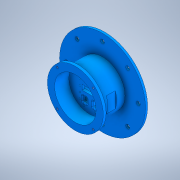
# Autodesk Inventor part: B-02
Saved by Autodesk Inventor 2021 (Build 250183000, 183)
## iProperties
Created: 2021-10-04
Part Number: B-02
Material: PETG
Document SubType Name: Modeling
Designer: Alcatraz
Density: 1.27 g/cm^3
Appearance: Genérico
Author: Alcatraz
Autodesk Inventor part; units mm, degrees
sketch "Boceto1" plane through (0, 0, 0) normal (0, 0, 1) x (1, 0, 0)
  line L0 (-16, -25) -> (16, -25)
  line L1 (16, -25) -> (16, 25)
  line L2 (16, 25) -> (-16, 25)
  line L3 (-16, 25) -> (-16, -25)
  line L4 (-16, -25) -> (16, 25) construction
  line L5 (16, -25) -> (-16, 25) construction
  circle A0 centre (0, 13.5) radius 6
  circle A1 centre (-8, -22.5) radius 1.1
  circle A2 centre (8, -22.5) radius 1.1
  circle A3 centre (13.5, -17) radius 1.1
  circle A4 centre (-13.5, -17) radius 1.1
  circle A5 centre (-13.5, -9) radius 1.1
  circle A6 centre (-13.5, -1) radius 1.1
  circle A7 centre (-13.5, 7) radius 1.1
  circle A8 centre (13.5, 7) radius 1.1
  circle A9 centre (13.5, -1) radius 1.1
  circle A10 centre (13.5, -9) radius 1.1
  line L6 (0, 1.85) -> (10.5, 1.85)
  line L7 (10.5, 1.85) -> (10.5, -5.15)
  line L8 (10.5, -5.15) -> (-10.5, -5.15)
  line L9 (-10.5, -5.15) -> (-10.5, 1.85)
  line L10 (-10.5, 1.85) -> (0, 1.85)
  line L11 (0, -25) -> (0, -15.266)
  line L12 (-7, -11.666) -> (-4.8, -11.666)
  line L13 (-7, -11.666) -> (-9.2, -11.666)
  line L14 (-10, -12.466) -> (-10, -18.066)
  line L15 (-9.2, -18.866) -> (-4.8, -18.866)
  line L16 (-4, -18.066) -> (-4, -12.466)
  line L17 (4, -15.266) -> (4, -18.066)
  line L18 (4.8, -18.866) -> (9.2, -18.866)
  line L19 (10, -18.066) -> (10, -12.466)
  line L20 (9.2, -11.666) -> (4.8, -11.666)
  line L21 (4, -15.266) -> (4, -12.466)
  arc A11 (-9.2, -11.666) -> (-10, -12.466) centre (-9.2, -12.466) ccw
  arc A12 (-4, -12.466) -> (-4.8, -11.666) centre (-4.8, -12.466) ccw
  arc A13 (-4.8, -18.866) -> (-4, -18.066) centre (-4.8, -18.066) ccw
  arc A14 (-10, -18.066) -> (-9.2, -18.866) centre (-9.2, -18.066) ccw
  arc A15 (4, -18.066) -> (4.8, -18.866) centre (4.8, -18.066) ccw
  arc A16 (9.2, -18.866) -> (10, -18.066) centre (9.2, -18.066) ccw
  arc A17 (10, -12.466) -> (9.2, -11.666) centre (9.2, -12.466) ccw
  arc A18 (4.8, -11.666) -> (4, -12.466) centre (4.8, -12.466) ccw
  point P0 (0, 0)
  dimension "d0" = 32
  dimension "d1" = 50
  dimension "d3" = 12
  dimension "d4" = 11.5
  dimension "d8" = 2.2
  dimension "d9" = 2.2
  dimension "d12" = 2.2
  dimension "d14" = 2.2
  dimension "d16" = 2.2
  dimension "d18" = 2.2
  dimension "BARRENOBASE" = 2.2
  dimension "d21" = 2.2
  dimension "d22" = 2.2
  dimension "d23" = 2.2
  dimension "d24" = 27
  dimension "d25" = 16
  dimension "d26" = 36
  dimension "d27" = 30.5
  dimension "d28" = 6.5
  dimension "DISTANCIAB" = 8
  dimension "d30" = 8
  dimension "d31" = 8
  dimension "d32" = 8
  dimension "d33" = 8
  dimension "d34" = 8
  dimension "d61" = 11.65
  dimension "d62" = 10.5
  dimension "d63" = 7
  dimension "d64" = 21
  dimension "d68" = 2.2
  dimension "d72" = 5.6
  dimension "d75" = 4
  dimension "d77" = 4.4
  dimension "d79" = 5.6
  dimension "d80" = 0.8
  dimension "d81" = 0.8
  dimension "d124" = 9.734
  dimension "d125" = 2.5
  constraints: 44 end point, 19 centre point, 16 point on circle, 6 tangent, 5 perpendicular, 4 horizontal, 3 midpoint, 2 parallel, 2 point on line, 2 vertical
  measures "d0" distance of L2.end L1.end
  measures "d1" distance of L1.end L0.end
  measures "d3" diameter of A0
  measures "d4" distance from line of L2 A0.centre
  measures "d8" diameter of A1
  measures "d9" diameter of A2
  measures "d12" diameter of A3
  measures "d14" diameter of A4
  measures "d16" diameter of A5
  measures "d18" diameter of A6
  measures "BARRENOBASE" diameter of A7
  measures "d21" diameter of A8
  measures "d22" diameter of A9
  measures "d23" diameter of A10
  measures "d24" distance of A3.centre A4.centre
  measures "d25" distance of A2.centre A1.centre
  measures "d26" vertical distance of A1.centre A0.centre
  measures "d27" vertical distance of A4.centre A0.centre
  measures "d28" vertical distance of A7.centre A0.centre
  measures "DISTANCIAB" distance of A9.centre A8.centre
  measures "d30" distance of A10.centre A9.centre
  measures "d31" distance of A3.centre A10.centre
  measures "d32" distance of A5.centre A4.centre
  measures "d33" distance of A5.centre A6.centre
  measures "d34" distance of A7.centre A6.centre
  measures "d61" distance of A0.centre L6.start
  measures "d62" distance of L6.start L6.end
  measures "d63" distance of L6.end L7.end
  measures "d64" distance of L7.end L8.end
  measures "d68" distance of L12.start L12.end
  measures "d72" distance of L14.start L14.end
  measures "d75" distance of L11.end L17.start
  measures "d77" distance of L18.start L18.end
  measures "d79" distance of L19.start L19.end
  measures "d80" radius of A11
  measures "d81" radius of A12
  measures "d124" distance of L11.start L11.end
  measures "d125" distance from line of L0 A1.centre
sketch "Boceto2" plane through (0, 0, 0) normal (0, 0, 1) x (1, 0, 0)
  circle A0 centre (0, 0) radius 29
  circle A1 centre (0, 0) radius 31.5
  dimension "DIAMETROINTERIOR" = 58
  dimension "d38" = 63
  constraints: 2 centre point, 2 coincident
  measures "DIAMETROINTERIOR" diameter of A0
  measures "d38" diameter of A1
extrude "Extrusión1" add sketch "Boceto2" against normal blind 38
ref_plane "Plano de trabajo1" through (0, 0, -24) normal (0, 0, 1) x (1, 0, 0)
sketch "Boceto3" plane through (0, 0, -24) normal (0, 0, 1) x (1, 0, 0)
  circle A0 centre (0, 0) radius 29
  dimension "d42" = 58
  constraints: 1 centre point, 1 coincident
  measures "d42" diameter of A0
extrude "Extrusión2" add sketch "Boceto3" along normal blind 4
sketch "Boceto4" plane through (0, 0, 0) normal (0, 0, 1) x (1, 0, 0)
  circle A0 centre (0, 0) radius 39
  circle A1 centre (0, 0) radius 31.5
  circle A2 centre (25.1022, 25.1024) radius 2
  circle A3 centre (25.1024, -25.1022) radius 2
  circle A4 centre (-25.1022, -25.1024) radius 2
  circle A5 centre (-25.1024, 25.1022) radius 2
  dimension "DIAMETROPESTAÑA" = 78
  dimension "d47" = 63
  dimension "d55" = 4
  dimension "d60" = 2
  dimension "d154" = 1.5
  dimension "d157" = 360
  constraints: 6 centre point, 4 coincident, 11 other
  measures "DIAMETROPESTAÑA" diameter of A0
  measures "d47" diameter of A1
  measures "d55" diameter of A2
extrude "Extrusión4" add sketch "Boceto4" against normal blind 4 contours A0 | A2 | A3 | A4 | A5
fillet "Empalme2" radius 2 1 edges at (-31.5, 0, -4)
extrude "Extrusión5" cut sketch "Boceto1" against normal blind 26 contours A0 | A1 | A2 | A3 | A4 | A5 | A6 | A7 | A8 | A9 | A10 | L6 L7 L8 L9 L10 | L12 A12 L16 A13 L15 A14 L14 A11 L13 | L21 A18 L20 A17 L19 A16 L18 A15 L17
fillet "Empalme3" radius 2 17 edges at (-6, 13.5, -20) (-4, -15.266, -20) (-4.2343, -18.6317, -20) (-7, -18.866, -20) (-9.7657, -18.6317, -20) (-10, -15.266, -20) (-9.7657, -11.9003, -20) (-7, -11.666, -20) (-4.2343, -11.9003, -20) (9.7657, -11.9003, -20) (10, -15.266, -20) (9.7657, -18.6317, -20) (7, -18.866, -20) (4.2343, -18.6317, -20) (4, -15.266, -20) (4.2343, -11.9003, -20) (7, -11.666, -20)
sketch "Boceto6" plane through (0, 0, -24) normal (0, 0, 1) x (1, 0, 0)
  circle A0 centre (0, 0) radius 60
  arc A1 (39, 0) -> (39, 0) centre (0, 0) ccw projected
  circle A2 centre (-50, 0) radius 2
  circle A3 centre (-35.3547, 35.356) radius 2
  circle A4 centre (0, 50) radius 2
  circle A5 centre (35.356, 35.3547) radius 2
  circle A6 centre (50, 0) radius 2
  circle A7 centre (35.3561, -35.3546) radius 2
  circle A8 centre (0, -50) radius 2
  circle A9 centre (-35.3566, -35.354) radius 2
  dimension "DIAMETROBASE" = 120
  dimension "d103" = 4
  dimension "d104" = 4
  dimension "d105" = 4
  dimension "d106" = 4
  dimension "d107" = 4
  dimension "d108" = 4
  dimension "d109" = 4
  dimension "d110" = 4
  dimension "RELACION" = 50
  dimension "d112" = 8
  dimension "d113" = 50
  dimension "d114" = 50
  dimension "d115" = 50
  dimension "d116" = 50
  dimension "d117" = 50
  dimension "d118" = 50
  dimension "d119" = 50
  constraints: 9 centre point, 1 coincident
  measures "DIAMETROBASE" diameter of A0
  measures "d103" diameter of A2
  measures "d104" diameter of A9
  measures "d105" diameter of A8
  measures "d106" diameter of A7
  measures "d107" diameter of A6
  measures "d108" diameter of A5
  measures "d109" diameter of A4
  measures "d110" diameter of A3
  measures "RELACION" distance of A5.centre point (0, 0)
  measures "d113" distance of point (0, 0) A4.centre
  measures "d114" distance of point (0, 0) A3.centre
  measures "d115" distance of A2.centre point (0, 0)
  measures "d116" distance of A9.centre point (0, 0)
  measures "d117" distance of point (0, 0) A8.centre
  measures "d118" distance of point (0, 0) A7.centre
  measures "d119" distance of point (0, 0) A6.centre
sketch "Boceto8" plane through (0, 0, -38) normal (0, 0, -1) x (-1, 0, 0)
  circle A0 centre (0, 0) radius 60
  circle A1 centre (0, 0) radius 45
  circle A2 centre (-50, 0) radius 2.75
  circle A3 centre (-35.3547, 35.356) radius 2.75
  circle A4 centre (0, 50) radius 2.75
  circle A5 centre (35.356, 35.3547) radius 2.75
  circle A6 centre (50, 0) radius 2.75
  circle A7 centre (35.3561, -35.3546) radius 2.75
  circle A8 centre (0, -50) radius 2.75
  circle A9 centre (-35.3566, -35.354) radius 2.75
  dimension "d126" = 120
  dimension "d127" = 5.5
  dimension "d128" = 5.5
  dimension "d129" = 5.5
  dimension "d130" = 5.5
  dimension "d131" = 5.5
  dimension "d132" = 5.5
  dimension "d133" = 5.5
  dimension "d134" = 5.5
  dimension "d135" = 50
  dimension "d136" = 7.25
  dimension "d137" = 50
  dimension "d138" = 50
  dimension "d139" = 50
  dimension "d140" = 50
  dimension "d141" = 50
  dimension "d142" = 50
  dimension "d143" = 50
  constraints: 10 centre point, 1 coincident
  measures "d126" diameter of A0
  measures "d127" diameter of A2
  measures "d128" diameter of A9
  measures "d129" diameter of A8
  measures "d130" diameter of A7
  measures "d131" diameter of A6
  measures "d132" diameter of A5
  measures "d133" diameter of A4
  measures "d134" diameter of A3
  measures "d135" distance of A5.centre point (0, 0)
  measures "d137" distance of point (0, 0) A4.centre
  measures "d138" distance of point (0, 0) A3.centre
  measures "d139" distance of A2.centre point (0, 0)
  measures "d140" distance of A9.centre point (0, 0)
  measures "d141" distance of point (0, 0) A8.centre
  measures "d142" distance of point (0, 0) A7.centre
  measures "d143" distance of point (0, 0) A6.centre
ref_plane "Plano de trabajo3" through (0, -31.5, 0) normal (0, 1, 0) x (-1, 0, 0)
sketch "Boceto9" plane through (0, -31.5, 0) normal (0, 1, 0) x (-1, 0, 0)
  line L0 (12.5, -26) -> (-12.5, -26)
  line L1 (-12.5, -26) -> (-12.5, -34)
  line L2 (-12.5, -34) -> (12.5, -34)
  line L3 (12.5, -34) -> (12.5, -26)
  line L4 (12.5, -26) -> (-12.5, -34) construction
  line L5 (-12.5, -26) -> (12.5, -34) construction
  point P0 (0, 0)
  point P1 (0, -30)
  dimension "d145" = 25
  dimension "d146" = 8
  constraints: 12 end point, 2 midpoint, 2 parallel, 1 horizontal, 1 perpendicular
  measures "d145" distance of L2.end L1.end
  measures "d146" distance of L1.end L0.end
extrude "Extrusión12" cut sketch "Boceto9" along normal blind 15
ref_plane "Plano de trabajo5" through (0, 0, -39) normal (0, 0, -1) x (-1, 0, 0)
hole "Agujero1" at (25.1022, 25.1024, 0) at (-25.1024, 25.1022, 0) at (-25.1022, -25.1024, 0) at (25.1024, -25.1022, 0) direction (0, 0, -1) diameter 2.85 depth 10.4 thread size "M3.5x0.6" class "6H" standard "ANSI Metric M Profile"
ref_plane "Plano de trabajo4" through (31.5, 0, 0) normal (1, 0, 0) x (0, 1, 0)
sketch "Boceto11" plane through (31.5, 0, 0) normal (1, 0, 0) x (0, 1, 0)
  line L0 (-17.5, -26.25) -> (17.5, -26.25)
  line L1 (17.5, -26.25) -> (17.5, -13.75)
  line L2 (17.5, -13.75) -> (-17.5, -13.75)
  line L3 (-17.5, -13.75) -> (-17.5, -26.25)
  line L4 (-29, -20) -> (29, -20) projected
  line L5 (-17.5, -26.25) -> (17.5, -13.75) construction
  line L6 (17.5, -26.25) -> (-17.5, -13.75) construction
  point P0 (0, 0)
  point P1 (0, -20)
  dimension "d166" = 35
  dimension "d167" = 12.5
  constraints: 12 end point, 3 midpoint, 2 parallel, 1 horizontal, 1 perpendicular
  measures "d166" distance of L2.end L1.end
  measures "d167" distance of L1.end L0.end
extrude "Extrusión14" cut sketch "Boceto11" against normal blind 2
extrude "Extrusión15" add sketch "Boceto8" along normal blind 3 contours A0 | A1
sketch "Boceto12" plane through (0, 0, -41) normal (0, 0, -1) x (-1, 0, 0)
  circle A0 centre (0, 0) radius 29
  dimension "d174" = 58
  constraints: 1 centre point, 1 coincident
  measures "d174" diameter of A0
extrude "Extrusión17" cut sketch "Boceto12" against normal blind 5
equation "\"d8\" = BARRENOBASE"
equation "\"d9\" = BARRENOBASE"
equation "\"d12\" = BARRENOBASE"
equation "\"d16\" = BARRENOBASE"
equation "\"d18\" = BARRENOBASE"
equation "\"d21\" = BARRENOBASE"
equation "\"d22\" = BARRENOBASE"
equation "\"d23\" = BARRENOBASE"
equation "\"d30\" = DISTANCIAB"
equation "\"d31\" = DISTANCIAB"
equation "\"d32\" = DISTANCIAB"
equation "\"d33\" = DISTANCIAB"
equation "\"d34\" = DISTANCIAB"
equation "\"d42\" = DIAMETROINTERIOR"
equation "\"d55\" = BARRENOEXTERIOR"
equation "\"d113\" = RELACION"
equation "\"d114\" = RELACION"
equation "\"d115\" = RELACION"
equation "\"d116\" = RELACION"
equation "\"d117\" = RELACION"
equation "\"d118\" = RELACION"
equation "\"d119\" = RELACION"
equation "\"d127\" = DiametroTornillos"
equation "\"d128\" = DiametroTornillos"
equation "\"d129\" = DiametroTornillos"
equation "\"d130\" = DiametroTornillos"
equation "\"d131\" = DiametroTornillos"
equation "\"d132\" = DiametroTornillos"
equation "\"d133\" = DiametroTornillos"
equation "\"d134\" = DiametroTornillos"
equation "\"d103\" = BARRENOEXTERIOR"
equation "\"d104\" = BARRENOEXTERIOR"
equation "\"d105\" = BARRENOEXTERIOR"
equation "\"d106\" = BARRENOEXTERIOR"
equation "\"d107\" = BARRENOEXTERIOR"
equation "\"d108\" = BARRENOEXTERIOR"
equation "\"d109\" = BARRENOEXTERIOR"
equation "\"d110\" = BARRENOEXTERIOR"
equation "\"d137\" = d135"
equation "\"d138\" = d135"
equation "\"d139\" = d135"
equation "\"d140\" = d135"
equation "\"d141\" = d135"
equation "\"d142\" = d135"
equation "\"d143\" = d135"
equation "\"BARRENOEXTERIOR\" = 4"
equation "\"DiametroTornillos\" = 5.5"
